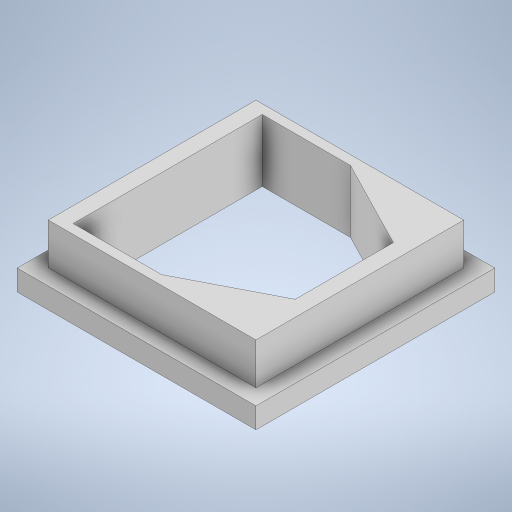
# Autodesk Inventor part: Adapter
Saved by Autodesk Inventor 2023 (Build 270158000, 158)
## iProperties
Created: 2022-05-02
Part Number: Adapter
Material: Generic
Document SubType Name: Modeling
Designer: cooki
Density: 1 g/cm^3
Appearance: Default
Author: cooki
Autodesk Inventor part; units mm, degrees
ref_plane "YZ Plane" through (0, 0, 0) normal (1, 0, 0) x (0, 1, 0)
ref_plane "XZ Plane" through (0, 0, 0) normal (0, 1, 0) x (-1, 0, 0)
ref_plane "XY Plane" through (0, 0, 0) normal (0, 0, 1) x (1, 0, 0)
sketch "Sketch1" plane through (0, 0, 0) normal (0, 1, 0) x (-1, 0, 0)
  line L0 (14.605, 14.605) -> (-14.605, 14.605)
  line L1 (-14.605, 14.605) -> (-14.605, -14.605)
  line L2 (-14.605, -14.605) -> (14.605, -14.605)
  line L3 (14.605, -14.605) -> (14.605, 14.605)
  point P0 (0, 0)
  point P1 (14.605, 0)
  point P2 (0, -14.605)
  dimension "d0" = 29.21
  dimension "d1" = 29.21
  constraints: 8 end point, 2 midpoint, 2 parallel, 1 horizontal, 1 horizontal alignment, 1 perpendicular, 1 vertical alignment
  measures "d0" distance of L2.end L1.end
  measures "d1" distance of L1.end L0.end
extrude "Extrusion1" add sketch "Sketch1" along normal blind 2.54
sketch "Sketch2" plane through (0, 2.54, 0) normal (0, 1, 0) x (1, 0, 0)
  line L0 (-12.7, -12.7) -> (12.7, -12.7)
  line L1 (12.7, -12.7) -> (12.7, 12.7)
  line L2 (12.7, 12.7) -> (-12.7, 12.7)
  line L3 (-12.7, 12.7) -> (-12.7, -12.7)
  point P0 (0, 0)
  point P1 (0, 12.7)
  point P2 (-12.7, 0)
  dimension "d4" = 25.4
  dimension "d5" = 25.4
  constraints: 8 end point, 2 midpoint, 2 parallel, 1 horizontal, 1 horizontal alignment, 1 perpendicular, 1 vertical alignment
  measures "d4" distance of L2.end L1.end
  measures "d5" distance of L1.end L0.end
extrude "Extrusion2" add sketch "Sketch2" along normal blind 5.08
sketch "Sketch3" plane through (0, 7.62, 0) normal (0, 1, 0) x (1, 0, 0)
  line L0 (0, 0) -> (0, 11.557)
  line L1 (0, 11.557) -> (0, -11.557)
  line L2 (0, -11.557) -> (0, -11.0469)
  line L3 (0, 0) -> (-10.795, 0)
  line L4 (-10.795, 0) -> (10.795, 0)
  line L5 (0, -11.557) -> (-10.795, -11.557)
  line L6 (-10.795, -11.557) -> (-10.795, 11.557)
  line L7 (-10.795, 11.557) -> (0, 11.557)
  line L8 (10.795, 0) -> (10.795, 6)
  line L9 (10.795, 6) -> (10.795, -6)
  line L10 (10.795, -6) -> (0, -11.557)
  line L11 (10.795, 6) -> (0, 11.557)
  dimension "d8" = 11.557
  dimension "d9" = 23.114
  dimension "d10" = 10.795
  dimension "d11" = 21.59
  dimension "d12" = 6
  dimension "d13" = 12
  constraints: 24 end point, 4 point on line, 2 horizontal, 2 perpendicular, 2 vertical
  measures "d8" distance of L0.start L0.end
  measures "d9" distance of L0.end L1.end
  measures "d10" distance of L0.start L3.end
  measures "d11" distance of L3.end L4.end
  measures "d12" distance of L4.end L8.end
  measures "d13" distance of L8.end L9.end
extrude "Extrusion3" cut sketch "Sketch3" against normal blind 25.4
body "Solid1"
